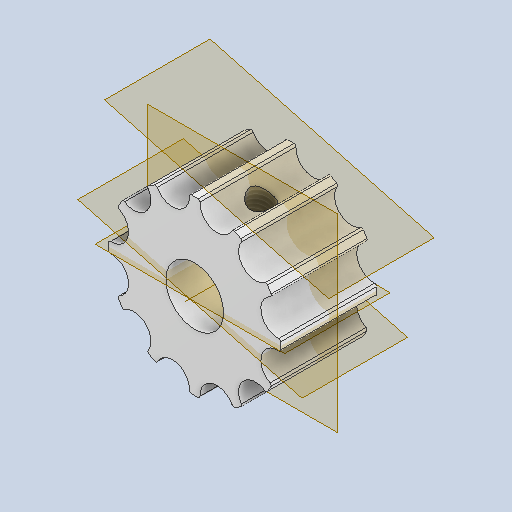
# Autodesk Inventor part: 12TBeltDisc
Saved by Autodesk Inventor 2022 (Build 260153000, 153)
## iProperties
Created: 2022-02-16
Part Number: 12TBeltDisc
Material: PBT-Kunststoff
Document SubType Name: Modeling
Designer: alexw
Mass: 2.173 g
Surface Area: 12.9079 cm^2
Volume: 1.65878 cm^3
Density: 1.31 g/cm^3
Appearance: Glatt - Weiß
Gear_Thick: 10,000 mm
GearDia: 19,099 mm
Dp_De_Diff_5: 1,140 mm
De: 21,140 mm
Dp: 22,280 mm
Author: alexw
Autodesk Inventor part; units mm, degrees
ref_plane "YZ Plane" through (0, 0, 0) normal (1, 0, 0) x (0, 1, 0)
ref_plane "XY Plane" through (0, 0, 0) normal (0, 0, 1) x (1, 0, 0)
sketch "Sketch1" plane through (0, 0, 0) normal (0, 0, 1) x (1, 0, 0)
  circle A0 centre (0, 0) radius 8.9793
  circle A1 centre (0, 0) radius 2.5
  circle A2 centre (0, 0) radius 9.5493 construction
  dimension "B_Gear_De" = 17.9586
  dimension "d1" = 5
  dimension "BigGear_D" = 19.0986
  constraints: 3 centre point, 3 coincident
  measures "B_Gear_De" diameter of A0
  measures "d1" diameter of A1
  measures "BigGear_D" diameter of A2
extrude "Extrusion1" add sketch "Sketch1" along normal blind 10 contours A0 | A1
ref_plane "Work Plane1" through (0, 0, 5) normal (0, 0, 1) x (1, 0, 0)
sketch "Sketch3" plane through (0, 0, 10) normal (0, 0, 1) x (1, 0, 0)
  circle A0 centre (0, 0) radius 8.9793 projected
  line L0 (0, 0) -> (0, 8.9793) construction
  circle A1 centre (0, 0) radius 8.9793 construction
  arc A2 (0.5522, 8.7622) -> (1.8649, 6.9597) centre (2.324, 8.6733) ccw
  arc A3 (-1.8649, 6.9597) -> (-0.5522, 8.7622) centre (-2.324, 8.6733) ccw
  arc A4 (2.324, 8.6733) -> (-2.324, 8.6733) centre (0, 0) ccw construction
  line L1 (-2.4715, 9.2239) -> (-1.8649, 6.9597) construction
  line L2 (2.4715, 9.2239) -> (1.8649, 6.9597) construction
  line L3 (0, 8.9793) -> (0, 9.5493) construction
  arc A5 (1.8649, 6.9597) -> (-1.8649, 6.9597) centre (0, 0) ccw construction
  circle A6 centre (0, 0) radius 9.5493 construction
  arc A7 (0.3605, 8.9721) -> (-0.3605, 8.9721) centre (0, 0) ccw
  arc A8 (-0.3605, 8.9721) -> (-0.5522, 8.7622) centre (-0.3524, 8.7722) ccw
  arc A9 (0.5522, 8.7622) -> (0.3605, 8.9721) centre (0.3524, 8.7722) ccw
  line L4 (0, 7.2052) -> (0, 8.9793) construction
  arc A10 (-0.5522, 8.7622) -> (-0.5734, 8.961) centre (-2.324, 8.6733) ccw construction
  arc A11 (0.5734, 8.961) -> (0.5522, 8.7622) centre (2.324, 8.6733) ccw construction
  line L5 (-1.8649, 6.9597) -> (0, 0) construction
  line L6 (0, 0) -> (1.8649, 6.9597) construction
  arc A12 (2.4715, 9.2239) -> (-2.4715, 9.2239) centre (0, 0) ccw construction
  circle A13 centre (0, 8.9793) radius 0.57 construction
  arc A14 (-5.0949, 5.0949) -> (-4.8593, 7.3122) centre (-6.3493, 6.3493) ccw
  arc A15 (-4.1739, 7.9503) -> (-4.7982, 7.5898) centre (0, 0) ccw
  arc A16 (-3.9029, 7.8644) -> (-4.1739, 7.9503) centre (-4.0809, 7.7732) ccw
  arc A17 (-3.9029, 7.8644) -> (-1.8649, 6.9597) centre (-2.324, 8.6733) ccw
  arc A18 (-4.7982, 7.5898) -> (-4.8593, 7.3122) centre (-4.6913, 7.4208) ccw
  arc A19 (-6.9597, 1.8649) -> (-7.8644, 3.9029) centre (-8.6733, 2.324) ccw
  arc A20 (-7.5898, 4.7982) -> (-7.9503, 4.1739) centre (0, 0) ccw
  arc A21 (-7.3122, 4.8593) -> (-7.5898, 4.7982) centre (-7.4208, 4.6913) ccw
  arc A22 (-7.3122, 4.8593) -> (-5.0949, 5.0949) centre (-6.3493, 6.3493) ccw
  arc A23 (-7.9503, 4.1739) -> (-7.8644, 3.9029) centre (-7.7732, 4.0809) ccw
  arc A24 (-6.9597, -1.8649) -> (-8.7622, -0.5522) centre (-8.6733, -2.324) ccw
  arc A25 (-8.9721, 0.3605) -> (-8.9721, -0.3605) centre (0, 0) ccw
  arc A26 (-8.7622, 0.5522) -> (-8.9721, 0.3605) centre (-8.7722, 0.3524) ccw
  arc A27 (-8.7622, 0.5522) -> (-6.9597, 1.8649) centre (-8.6733, 2.324) ccw
  arc A28 (-8.9721, -0.3605) -> (-8.7622, -0.5522) centre (-8.7722, -0.3524) ccw
  arc A29 (-5.0949, -5.0949) -> (-7.3122, -4.8593) centre (-6.3493, -6.3493) ccw
  arc A30 (-7.9503, -4.1739) -> (-7.5898, -4.7982) centre (0, 0) ccw
  arc A31 (-7.8644, -3.9029) -> (-7.9503, -4.1739) centre (-7.7732, -4.0809) ccw
  arc A32 (-7.8644, -3.9029) -> (-6.9597, -1.8649) centre (-8.6733, -2.324) ccw
  arc A33 (-7.5898, -4.7982) -> (-7.3122, -4.8593) centre (-7.4208, -4.6913) ccw
  arc A34 (-1.8649, -6.9597) -> (-3.9029, -7.8644) centre (-2.324, -8.6733) ccw
  arc A35 (-4.7982, -7.5898) -> (-4.1739, -7.9503) centre (0, 0) ccw
  arc A36 (-4.8593, -7.3122) -> (-4.7982, -7.5898) centre (-4.6913, -7.4208) ccw
  arc A37 (-4.8593, -7.3122) -> (-5.0949, -5.0949) centre (-6.3493, -6.3493) ccw
  arc A38 (-4.1739, -7.9503) -> (-3.9029, -7.8644) centre (-4.0809, -7.7732) ccw
  arc A39 (1.8649, -6.9597) -> (0.5522, -8.7622) centre (2.324, -8.6733) ccw
  arc A40 (-0.3605, -8.9721) -> (0.3605, -8.9721) centre (0, 0) ccw
  arc A41 (-0.5522, -8.7622) -> (-0.3605, -8.9721) centre (-0.3524, -8.7722) ccw
  arc A42 (-0.5522, -8.7622) -> (-1.8649, -6.9597) centre (-2.324, -8.6733) ccw
  arc A43 (0.3605, -8.9721) -> (0.5522, -8.7622) centre (0.3524, -8.7722) ccw
  arc A44 (5.0949, -5.0949) -> (4.8593, -7.3122) centre (6.3493, -6.3493) ccw
  arc A45 (4.1739, -7.9503) -> (4.7982, -7.5898) centre (0, 0) ccw
  arc A46 (3.9029, -7.8644) -> (4.1739, -7.9503) centre (4.0809, -7.7732) ccw
  arc A47 (3.9029, -7.8644) -> (1.8649, -6.9597) centre (2.324, -8.6733) ccw
  arc A48 (4.7982, -7.5898) -> (4.8593, -7.3122) centre (4.6913, -7.4208) ccw
  arc A49 (6.9597, -1.8649) -> (7.8644, -3.9029) centre (8.6733, -2.324) ccw
  arc A50 (7.5898, -4.7982) -> (7.9503, -4.1739) centre (0, 0) ccw
  arc A51 (7.3122, -4.8593) -> (7.5898, -4.7982) centre (7.4208, -4.6913) ccw
  arc A52 (7.3122, -4.8593) -> (5.0949, -5.0949) centre (6.3493, -6.3493) ccw
  arc A53 (7.9503, -4.1739) -> (7.8644, -3.9029) centre (7.7732, -4.0809) ccw
  arc A54 (6.9597, 1.8649) -> (8.7622, 0.5522) centre (8.6733, 2.324) ccw
  arc A55 (8.9721, -0.3605) -> (8.9721, 0.3605) centre (0, 0) ccw
  arc A56 (8.7622, -0.5522) -> (8.9721, -0.3605) centre (8.7722, -0.3524) ccw
  arc A57 (8.7622, -0.5522) -> (6.9597, -1.8649) centre (8.6733, -2.324) ccw
  arc A58 (8.9721, 0.3605) -> (8.7622, 0.5522) centre (8.7722, 0.3524) ccw
  arc A59 (5.0949, 5.0949) -> (7.3122, 4.8593) centre (6.3493, 6.3493) ccw
  arc A60 (7.9503, 4.1739) -> (7.5898, 4.7982) centre (0, 0) ccw
  arc A61 (7.8644, 3.9029) -> (7.9503, 4.1739) centre (7.7732, 4.0809) ccw
  arc A62 (7.8644, 3.9029) -> (6.9597, 1.8649) centre (8.6733, 2.324) ccw
  arc A63 (7.5898, 4.7982) -> (7.3122, 4.8593) centre (7.4208, 4.6913) ccw
  arc A64 (1.8649, 6.9597) -> (3.9029, 7.8644) centre (2.324, 8.6733) ccw
  arc A65 (4.7982, 7.5898) -> (4.1739, 7.9503) centre (0, 0) ccw
  arc A66 (4.8593, 7.3122) -> (4.7982, 7.5898) centre (4.6913, 7.4208) ccw
  arc A67 (4.8593, 7.3122) -> (5.0949, 5.0949) centre (6.3493, 6.3493) ccw
  arc A68 (4.1739, 7.9503) -> (3.9029, 7.8644) centre (4.0809, 7.7732) ccw
  point P0 (-0.3605, 8.9721)
  point P1 (-0.3605, 8.9721)
  point P2 (0, 9.5493)
  point P3 (-4.4896, 7.7763)
  point P4 (-7.7763, 4.4896)
  point P5 (-8.9793, 0)
  point P6 (-7.7763, -4.4896)
  point P7 (-4.4896, -7.7763)
  point P8 (0, -8.9793)
  point P9 (4.4896, -7.7763)
  point P10 (7.7763, -4.4896)
  point P11 (8.9793, 0)
  point P12 (7.7763, 4.4896)
  point P13 (4.4896, 7.7763)
  point P14 (1.8649, 6.9597)
  point P15 (4.1739, 7.9503)
  point P16 (-1.8649, 6.9597)
  point P17 (-4.1739, 7.9503)
  point P18 (-5.0949, 5.0949)
  point P19 (-4.7982, 7.5898)
  point P20 (-7.5898, 4.7982)
  point P21 (-6.9597, 1.8649)
  point P22 (-7.9503, 4.1739)
  point P23 (-8.9721, 0.3605)
  point P24 (-6.9597, -1.8649)
  point P25 (-8.9721, -0.3605)
  point P26 (-7.9503, -4.1739)
  point P27 (-7.5898, -4.7982)
  point P28 (-4.7982, -7.5898)
  point P29 (-1.8649, -6.9597)
  point P30 (-4.1739, -7.9503)
  point P31 (-0.3605, -8.9721)
  point P32 (1.8649, -6.9597)
  point P33 (0.3605, -8.9721)
  point P34 (4.1739, -7.9503)
  point P35 (4.7982, -7.5898)
  point P36 (7.5898, -4.7982)
  point P37 (6.9597, -1.8649)
  point P38 (7.9503, -4.1739)
  point P39 (8.9721, -0.3605)
  point P40 (6.9597, 1.8649)
  point P41 (8.9721, 0.3605)
  point P42 (7.9503, 4.1739)
  point P43 (7.5898, 4.7982)
  point P44 (4.7982, 7.5898)
  dimension "d33" = 0.2
  dimension "d56" = 5
  dimension "d59" = 360
  constraints: 151 point on circle, 65 centre point, 14 end point, 7 coincident, 5 line through centre, 4 concentric, 4 point on line, 4 tangent, 2 equal radius, 2 vertical, 2 vertical alignment, 1 collinear, 214 other
  measures "d33" radius of A8
extrude "Zahnprofil" cut sketch "Sketch3" against normal through all contours A58 A54 A62 A61 A0 | A0 A53 A49 A57 A56 | A63 A59 A67 A66 A0 | A0 A48 A44 A52 A51 | A68 A64 A2 A9 A0 | A0 A43 A39 A47 A46 | A8 A3 A17 A16 A0 | A0 A38 A34 A42 A41 | A18 A14 A22 A21 A0 | A0 A33 A29 A37 A36 | A23 A19 A27 A26 A0 | A0 A28 A24 A32 A31
sketch "Skizze6" plane through (0, 0, 10) normal (0, 0, 1) x (1, 0, 0)
  circle A0 centre (0, 0) radius 3
  dimension "d50" = 6
  constraints: 1 centre point, 1 coincident
  measures "d50" diameter of A0
extrude "Extrusion4" cut sketch "Skizze6" against normal blind 10
ref_plane "Arbeitsebene3" through (2.7832, 10.387, 10) normal (0.258819, 0.9659258, 0) x (0, 0, -1)
ref_plane "Arbeitsebene2" through (0, 0, 10) normal (0.258819, 0.9659258, 0) x (0, 0, -1)
sketch "Skizze7" plane through (2.7832, 10.387, 10) normal (0.258819, 0.9659258, 0) x (0, 0, -1)
  line L0 (10, 1.7345) -> (10, -1.7345) construction
  line L1 (0, 1.7345) -> (10, 1.7345) construction
  line L2 (0, -1.7345) -> (0, 1.7345) construction
  line L3 (0, -1.7345) -> (10, -1.7345) construction
  line L4 (0, -1.7345) -> (10, -1.7345) construction
  line L5 (5, -1.7345) -> (5, 1.7345) construction
  line L6 (0, 1.7345) -> (10, 1.7345) construction
  point P0 (10, 0)
  point P1 (5, 0)
  constraints: 3 midpoint, 2 end point
hole "Bohrung2" at (2.7832, 10.387, 5) direction (-0.258819, -0.9659258, 0) diameter 2.459 end up to face face through (0, 0, 10) facing (0, 0, -1) round with radius 3 far side no thread size "M3x0.5" class "6H" standard "ISO Metric profile"
ref_plane "Arbeitsebene4" through (0, 0, 5) normal (0, 0, 1) x (1, 0, 0)
equation "\"Teilung\" = 5"
equation "\"GearDia\" = 19.09859"
equation "\"Dp_De_Diff_5\" = 1.14"
equation "\"De\" = 21.14"
equation "\"Dp\" = 22.28"
body "Solid1"
